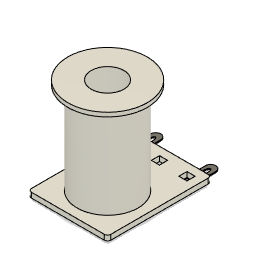
Appearing Post A-17932 (Autodesk Fusion 360 archive; units mm, degrees)
design "AE-27-1200 Coil"
Autodesk Fusion 360 part; units mm, degrees
sketch "Sketch1" plane through (0, 0, 0) normal (0, 1, 0) x (1, 0, 0) in component "Winding"
  circle A0 centre (0, 0) radius 11.9062
  circle A1 centre (0, 0) radius 6.35
  circle A2 centre (0, 0) radius 7.1437
  dimension "d1" = 23.8125
  dimension "d2" = 12.7
  dimension "d3" = 0.7937
  constraint coincident A0.centre A1.centre
  constraint concentric A0 A1
  constraint concentric A1 A2
  measures "d1" diameter of A0
  measures "d2" diameter of A1
  measures "d3" distance of A1 A2
extrude "Extrude1" add sketch "Sketch1" along normal blind 35.7188 contours A0 makes body 1 in component "Winding"
sketch "Sketch1 (2)" plane through (0, 35.7188, 0) normal (0, 1, 0) x (-1, 0, 0) in component "Coil Body"
  circle A0 centre (0, 0) radius 7.1437
  circle A1 centre (0, 0) radius 11.9062
  circle A2 centre (-50.8, 0) radius 15.4781
  circle A3 centre (-50.8, 0) radius 6.35
  circle A4 centre (-50.8, 0) radius 7.1437
  point P0 (-50.8, 0)
  dimension "d6" = 30.9563
  dimension "d7" = 12.7
  dimension "d8" = 0.7937
  constraint coincident P0 A2.centre
  constraint concentric A2 A3
  constraint concentric A3 A4
  measures "d6" diameter of A2
  measures "d7" diameter of A3
  measures "d8" distance of A3 A4
extrude "Extrude1'" add sketch "Sketch1 (2)" against normal blind 35.7188 separate body contours A4 makes body 2 in component "Coil Body"
extrude "Extrude2" add sketch "Sketch1 (2)" along normal blind 1.5875 contours A2 | A4 bodies 2 in component "Coil Body"
sketch "Sketch2" plane through (0, 0, 0) normal (0, -1, 0) x (1, 0, 0) in component "Coil Body"
  circle A0 centre (50.8, 0) radius 6.35
  circle A1 centre (50.8, 0) radius 7.1438
  line L0 (50.8, 0) -> (50.8, 6.35)
  circle A2 centre (50.8, 0) radius 15.4781
  line L1 (50.8, 6.35) -> (50.8, 15.4781)
  line L2 (50.8, 15.4781) -> (65.0081, 15.4781)
  line L3 (50.8, 15.4781) -> (36.5919, 15.4781)
  line L4 (35.3219, 14.2081) -> (35.3219, -23.7331)
  line L5 (36.5919, -25.0031) -> (65.0081, -25.0031)
  line L6 (66.2781, -23.7331) -> (66.2781, 14.2081)
  arc A3 (35.3219, -23.7331) -> (36.5919, -25.0031) centre (36.5919, -23.7331) ccw
  arc A4 (65.0081, -25.0031) -> (66.2781, -23.7331) centre (65.0081, -23.7331) ccw
  arc A5 (66.2781, 14.2081) -> (65.0081, 15.4781) centre (65.0081, 14.2081) ccw
  arc A6 (36.5919, 15.4781) -> (35.3219, 14.2081) centre (36.5919, 14.2081) ccw
  point P0 (66.2781, 15.4781)
  point P1 (35.3219, 15.4781)
  point P2 (35.3219, -25.0031)
  point P3 (66.2781, -25.0031)
  dimension "d13" = 15.4781
  dimension "d14" = 15.4781
  dimension "d15" = 40.4812
  dimension "d16" = 30.9563
  dimension "d19" = 1.27
  dimension "d20" = 1.27
  dimension "d21" = 1.27
  dimension "d22" = 1.27
  constraint coincident A0.centre A1.centre
  constraint coincident A0 L0.end
  constraint coincident A2 L1.end
  constraint parallel L0 L1
  constraint perpendicular L1 L2
  constraint perpendicular L1 L3
  constraint perpendicular L3 L4
  constraint perpendicular L4 L5
  constraint coincident P2 L4
  constraint coincident P2 L5
  constraint tangent L4 A3
  constraint tangent L5 A3
  constraint coincident P3 L5
  constraint coincident P3 L6
  constraint tangent L5 A4
  constraint tangent L6 A4
  constraint coincident P0 L2
  constraint coincident P0 L6
  constraint tangent L2 A5
  constraint tangent L6 A5
  constraint coincident P1 L3
  constraint coincident P1 L4
  constraint tangent L3 A6
  constraint tangent L4 A6
  measures "d13" distance of L1.end P0
  measures "d14" distance of L1.end P1
  measures "d15" distance of P1 P2
  measures "d16" distance of P2 P3
  measures "d19" radius of A3
  measures "d20" radius of A4
  measures "d21" radius of A5
  measures "d22" radius of A6
extrude "Extrude3" add sketch "Sketch2" along normal blind 1.9844 contours A1 | A2 | A2 L4 L5 L6 A3 A4 | A2 L2 L6 A5 | A2 L3 L4 A6 bodies 2 in component "Coil Body"
sketch "Sketch3" plane through (0, -1.9844, 0) normal (0, -1, 0) x (1, 0, 0) in component "Coil Body"
  circle A0 centre (50.8, 0) radius 6.35
  line L0 (65.0081, 15.4781) -> (36.5919, 15.4781)
  arc A1 (36.5919, 15.4781) -> (35.3219, 14.2081) centre (36.5919, 14.2081) ccw
  line L1 (35.3219, 14.2081) -> (35.3219, -23.7331)
  arc A2 (35.3219, -23.7331) -> (36.5919, -25.0031) centre (36.5919, -23.7331) ccw
  line L2 (36.5919, -25.0031) -> (65.0081, -25.0031)
  arc A3 (65.0081, -25.0031) -> (66.2781, -23.7331) centre (65.0081, -23.7331) ccw
  line L3 (66.2781, -23.7331) -> (66.2781, 14.2081)
  arc A4 (66.2781, 14.2081) -> (65.0081, 15.4781) centre (65.0081, 14.2081) ccw
  line L4 (35.3219, -25.0031) -> (38.4969, -25.0031)
  line L5 (38.4969, -25.0031) -> (38.4969, -21.8281)
  line L6 (38.4969, -21.8281) -> (41.6719, -21.8281)
  line L7 (41.6719, -21.8281) -> (41.6719, -18.6531)
  line L8 (41.6719, -18.6531) -> (38.4969, -18.6531)
  line L9 (38.4969, -18.6531) -> (38.4969, -21.8281)
  line L10 (66.2781, -25.0031) -> (63.1031, -25.0031)
  line L11 (63.1031, -25.0031) -> (63.1031, -21.8281)
  line L12 (63.1031, -21.8281) -> (59.9281, -21.8281)
  line L13 (59.9281, -21.8281) -> (59.9281, -18.6531)
  line L14 (59.9281, -18.6531) -> (63.1031, -18.6531)
  line L15 (63.1031, -18.6531) -> (63.1031, -21.8281)
  line L16 (50.8, -25.0031) -> (52.3875, -25.0031)
  line L17 (52.3875, -25.0031) -> (52.3875, -21.8281)
  line L18 (52.3875, -21.8281) -> (49.2125, -21.8281)
  line L19 (49.2125, -21.8281) -> (49.2125, -18.6531)
  line L20 (49.2125, -18.6531) -> (52.3875, -18.6531)
  line L21 (52.3875, -18.6531) -> (52.3875, -21.8281)
  dimension "d23" = 3.175
  dimension "d24" = 3.175
  dimension "d25" = 3.175
  dimension "d26" = 3.175
  dimension "d27" = 3.175
  dimension "d28" = 3.175
  dimension "d29" = 3.175
  dimension "d30" = 3.175
  dimension "d31" = 1.5875
  dimension "d32" = 3.175
  dimension "d33" = 3.175
  dimension "d34" = 3.175
  constraint perpendicular L1 L4
  constraint perpendicular L4 L5
  constraint horizontal L6
  constraint vertical L7
  constraint horizontal L8
  constraint vertical L9
  constraint parallel L2 L10
  constraint perpendicular L10 L11
  constraint horizontal L12
  constraint vertical L13
  constraint horizontal L14
  constraint vertical L15
  constraint midpoint L2 L16.start
  constraint parallel L2 L16
  constraint perpendicular L2 L17
  constraint horizontal L18
  constraint vertical L19
  constraint horizontal L20
  constraint vertical L21
  measures "d23" distance of L4.start L4.end
  measures "d24" distance of L4.end L5.end
  measures "d25" distance of L5.end L6.end
  measures "d26" distance of L5.end L8.end
  measures "d27" distance of L10.start L10.end
  measures "d28" distance of L10.end L11.end
  measures "d29" distance of L11.end L12.end
  measures "d30" distance of L11.end L14.end
  measures "d31" distance of L16.start L16.end
  measures "d32" distance of L16.end L17.end
  measures "d33" distance of L17.end L18.end
  measures "d34" distance of L17.end L20.end
extrude "Extrude4" cut sketch "Sketch3" against normal blind 1.9844 contours L6 L7 L8 L9 | L12 L13 L14 L15 | L18 L19 L20 L21 bodies 2 in component "Coil Body"
sketch "Sketch4" plane through (0, -1.9844, 0) normal (0, -1, 0) x (1, 0, 0) in component "Coil Body"
  line L0 (49.2125, -21.8281) -> (49.2125, -18.6531)
  line L1 (49.2125, -18.6531) -> (52.3875, -18.6531)
  line L2 (52.3875, -18.6531) -> (52.3875, -21.8281)
  line L3 (52.3875, -21.8281) -> (49.2125, -21.8281)
  line L4 (41.6719, -21.8281) -> (38.4969, -21.8281)
  line L5 (38.4969, -21.8281) -> (38.4969, -18.6531)
  line L6 (38.4969, -18.6531) -> (41.6719, -18.6531)
  line L7 (41.6719, -18.6531) -> (41.6719, -21.8281)
  line L8 (59.9281, -21.8281) -> (59.9281, -18.6531)
  line L9 (59.9281, -18.6531) -> (63.1031, -18.6531)
  line L10 (63.1031, -18.6531) -> (63.1031, -21.8281)
  line L11 (63.1031, -21.8281) -> (59.9281, -21.8281)
  circle A0 centre (50.8, 0) radius 6.35
  line L12 (65.0081, 15.4781) -> (36.5919, 15.4781)
  arc A1 (36.5919, 15.4781) -> (35.3219, 14.2081) centre (36.5919, 14.2081) ccw
  line L13 (35.3219, 14.2081) -> (35.3219, -23.7331)
  arc A2 (35.3219, -23.7331) -> (36.5919, -25.0031) centre (36.5919, -23.7331) ccw
  line L14 (36.5919, -25.0031) -> (65.0081, -25.0031)
  arc A3 (65.0081, -25.0031) -> (66.2781, -23.7331) centre (65.0081, -23.7331) ccw
  line L15 (66.2781, -23.7331) -> (66.2781, 14.2081)
  arc A4 (66.2781, 14.2081) -> (65.0081, 15.4781) centre (65.0081, 14.2081) ccw
  line L16 (50.8, -25.0031) -> (53.975, -25.0031)
  line L17 (50.8, -25.0031) -> (47.625, -25.0031)
  line L18 (47.625, -25.0031) -> (43.2594, -25.0031)
  line L19 (43.2594, -25.0031) -> (43.2594, -16.2719)
  line L20 (43.2594, -16.2719) -> (47.625, -16.2719)
  line L21 (47.625, -16.2719) -> (47.625, -25.0031)
  line L22 (53.975, -25.0031) -> (58.3406, -25.0031)
  line L23 (58.3406, -25.0031) -> (58.3406, -16.2719)
  line L24 (58.3406, -16.2719) -> (53.975, -16.2719)
  line L25 (53.975, -16.2719) -> (53.975, -25.0031)
  dimension "d37" = 3.175
  dimension "d40" = 3.175
  dimension "d41" = 8.7313
  dimension "d42" = 4.3656
  dimension "d43" = 8.7313
  dimension "d44" = 4.3656
  constraint midpoint L14 L16.start
  constraint parallel L14 L16
  constraint parallel L16 L17
  constraint horizontal L18
  constraint vertical L19
  constraint horizontal L20
  constraint vertical L21
  constraint horizontal L22
  constraint vertical L23
  constraint horizontal L24
  constraint vertical L25
  measures "d37" distance of L16.start L16.end
  measures "d40" distance of L16.start L17.end
  measures "d41" distance of L17.end L20.end
  measures "d42" distance of L17.end L18.end
  measures "d43" distance of L16.end L24.end
  measures "d44" distance of L16.end L22.end
extrude "Extrude5" add sketch "Sketch4" along normal blind 1.1906 contours L14 L22 L23 L24 L25 | L14 L18 L19 L20 L21 bodies 2 in component "Coil Body"
sketch "Sketch1 (3)" plane through (0, 0, 0) normal (0, 1, 0) x (1, 0, 0) in component "Solder Tab"
  line L0 (12.6083, 21.8281) -> (9.4333, 21.8281)
  line L1 (12.5671, 18.6531) -> (12.6083, 21.8281)
  line L2 (9.3921, 18.6531) -> (12.5671, 18.6531)
  line L3 (9.4333, 21.8281) -> (9.3921, 18.6531)
  circle A0 centre (11.0204, 20.2395) radius 2.3813
  line L4 (11.0208, 21.8281) -> (9.0364, 21.8281)
  line L5 (9.0364, 21.8281) -> (13.0052, 21.8281)
  line L6 (9.0364, 21.8281) -> (9.0364, 21.5564)
  line L7 (13.0052, 21.8281) -> (13.0052, 21.7834)
  line L8 (13.0052, 21.7834) -> (13.0052, 21.5552)
  line L9 (9.0364, 29.4349) -> (9.0364, 21.8281)
  line L10 (13.0052, 21.8281) -> (13.0052, 29.4349)
  arc A1 (13.0052, 29.4349) -> (9.0364, 29.4349) centre (11.0208, 29.4349) ccw
  ellipse E0 centre (10.9794, 27.6022) end of major axis (10.9437, 25.8229) minor radius 0.7677
  line L11 (11.015, 29.3815) -> (10.9437, 25.8229)
  line L12 (10.2118, 27.6176) -> (11.7469, 27.5868)
  line L13 (9.0364, 29.4349) -> (13.0052, 29.4349)
  dimension "d47" = 4.7625
  dimension "d48" = 1.9844
  dimension "d49" = 3.9688
  dimension "d52" = 3.9688
  constraint midpoint L0 L4.start
  constraint parallel L0 L4
  constraint horizontal L4
  constraint horizontal L5
  constraint coincident A0 L6.end
  constraint perpendicular L5 L6
  constraint perpendicular L5 L7
  constraint coincident A0 L8.end
  constraint perpendicular L5 L8
  constraint vertical L10
  constraint tangent L10 A1
  constraint tangent L9 A1
  constraint coincident E0 L11.start
  constraint coincident E0 L11.end
  constraint coincident E0 L12.start
  constraint coincident E0 L12.end
  measures "d47" diameter of A0
  measures "d48" distance of L4.start L4.end
  measures "d49" distance of L4.end L5.end
  measures "d52" horizontal distance of L9.start L10.end
extrude "Extrude1''" add sketch "Sketch1 (3)" along normal blind 0.3969 separate body contours L1 L2 L3 A0 L4 L5 | L0 A0 L4 L5 | A0 L5 L7 L8 | A0 L4 L5 L9 L10 L13 | A0 L4 L5 L6 | A1 L13 makes body 3 in component "Solder Tab"
component "Winding" placed x (1, 0, 0) y (0, 1, 0) z (0, 0, 1) at (0, 0, 0)
component "Coil Body" placed x (1, 0, 0) y (0, 1, 0) z (0, 0, 1) at (-50.8, 0, 0)
component "Solder Tab" placed x (1, 0, 0) y (0, 1, 0) z (0, 0, 1) at (-0.264, -2.3813, 0)
component "Solder Tab" placed x (1, 0, 0) y (0, 1, 0) z (0, 0, 1) at (-21.6952, -2.3812, 0)
equation "d1 = ( 15 / 16 ) * 1 in"
equation "d2 = ( 1 / 2 ) * 1 in"
equation "d3 = ( 1 / 32 ) * 1 in"
equation "d4 = 1 13/32\""
equation "d6 = 1 7/32\""
equation "d7 = ( 1 / 2 ) * 1 in"
equation "d8 = ( 1 / 32 ) * 1 in"
equation "d9 = -1 13/32\""
equation "d11 = ( 1 / 16 ) * 1 in"
equation "d13 = ( 39 / 64 ) * 1 in"
equation "d14 = ( 39 / 64 ) * 1 in"
equation "d15 = 1 19/32\""
equation "d16 = 1 7/32\""
equation "d17 = ( 5 / 64 ) * 1 in"
equation "d23 = ( 1 / 8 ) * 1 in"
equation "d24 = ( 1 / 8 ) * 1 in"
equation "d25 = ( 1 / 8 ) * 1 in"
equation "d26 = ( 1 / 8 ) * 1 in"
equation "d27 = ( 1 / 8 ) * 1 in"
equation "d28 = ( 1 / 8 ) * 1 in"
equation "d29 = ( 1 / 8 ) * 1 in"
equation "d30 = ( 1 / 8 ) * 1 in"
equation "d31 = ( 1 / 16 ) * 1 in"
equation "d32 = ( 1 / 8 ) * 1 in"
equation "d33 = ( 1 / 8 ) * 1 in"
equation "d34 = ( 1 / 8 ) * 1 in"
equation "d35 = ( -5 / 64 ) * 1 in"
equation "d37 = ( 1 / 8 ) * 1 in"
equation "d40 = ( 1 / 8 ) * 1 in"
equation "d41 = ( 11 / 32 ) * 1 in"
equation "d42 = ( 11 / 64 ) * 1 in"
equation "d43 = ( 11 / 32 ) * 1 in"
equation "d44 = ( 11 / 64 ) * 1 in"
equation "d45 = ( 3 / 64 ) * 1 in"
equation "d47 = ( 3 / 16 ) * 1 in"
equation "d48 = ( 5 / 64 ) * 1 in"
equation "d49 = ( 5 / 32 ) * 1 in"
equation "d52 = ( 5 / 32 ) * 1 in"
equation "d53 = ( 1 / 64 ) * 1 in"

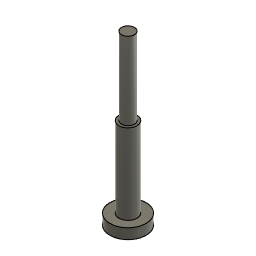
design "Appearing Post Armature"
Autodesk Fusion 360 part; units mm, degrees
sketch "Sketch1" plane through (0, 0, 0) normal (0, 1, 0) x (1, 0, 0)
  circle A0 centre (0, 0) radius 11.1125
  circle A1 centre (0, 0) radius 5.5562
  circle A2 centre (0, 0) radius 3.9688
  dimension "d1" = 22.225
  dimension "d2" = 11.1125
  dimension "d3" = 7.9375
  constraint coincident A0.centre A1.centre
  constraint concentric A0 A1
  constraint concentric A1 A2
  measures "d1" diameter of A0
  measures "d2" diameter of A1
  measures "d3" diameter of A2
extrude "Extrude1" add sketch "Sketch1" along normal blind 103.1875 contours A2
extrude "Extrude2" add sketch "Sketch1" along normal blind 55.5625 contours A1
extrude "Extrude3" add sketch "Sketch1" along normal blind 6.35 contours A0
equation "d1 = ( 7 / 8 ) * 1 in"
equation "d2 = ( 7 / 16 ) * 1 in"
equation "d3 = ( 5 / 16 ) * 1 in"
equation "d4 = 4 1/16\""
equation "d6 = 2 3/16\""
equation "d8 = ( 1 / 4 ) * 1 in"

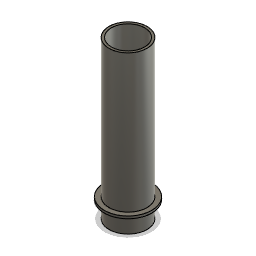
design "Coil Sleeve 2 1/16 With Lip"
Autodesk Fusion 360 part; units mm, degrees
sketch "Sketch1" plane through (0, 0, 0) normal (0, 1, 0) x (1, 0, 0)
  circle A0 centre (0, 0) radius 6.35
  circle A1 centre (0, 0) radius 5.5563
  circle A2 centre (0, 0) radius 7.9375
  dimension "d1" = 12.7
  dimension "d2" = 0.7937
  dimension "d3" = 15.875
  constraint coincident A0.centre A1.centre
  measures "d1" diameter of A0
  measures "d2" distance of A0 A1
  measures "d3" diameter of A2
extrude "Extrude1" add sketch "Sketch1" along normal blind 46.0375 contours A0
extrude "Extrude2" add sketch "Sketch1" against normal blind 6.35 contours A0
extrude "Extrude3" add sketch "Sketch1" against normal blind 0.7937 contours A2
equation "d1 = ( 1 / 2 ) * 1 in"
equation "d2 = ( 1 / 32 ) * 1 in"
equation "d3 = ( 5 / 8 ) * 1 in"
equation "d4 = 1 13/16\""
equation "d6 = ( -1 / 4 ) * 1 in"
equation "d8 = ( -1 / 32 ) * 1 in"
